Autodesk Fusion 360 part; units mm, degrees
(part 4 of 9)
  arc A178 (-216.55, 3.525) -> (-215.55, 2.525) centre (-215.55, 3.525) ccw
  line L174 (-216.55, 3.525) -> (-216.55, 15.525)
  arc A179 (-215.55, 16.525) -> (-216.55, 15.525) centre (-215.55, 15.525) ccw
  line L175 (-215.55, 16.525) -> (-203.55, 16.525)
  arc A180 (-202.55, 15.525) -> (-203.55, 16.525) centre (-203.55, 15.525) ccw
  line L176 (-243.0312, 53.625) -> (-243.0312, 41.625)
  arc A181 (-244.0312, 40.625) -> (-243.0313, 41.625) centre (-244.0313, 41.625) ccw
  line L177 (-244.0312, 40.625) -> (-256.0312, 40.625)
  arc A182 (-257.0312, 41.625) -> (-256.0312, 40.625) centre (-256.0312, 41.625) ccw
  line L178 (-257.0312, 41.625) -> (-257.0312, 53.625)
  arc A183 (-256.0312, 54.625) -> (-257.0312, 53.625) centre (-256.0312, 53.625) ccw
  line L179 (-256.0312, 54.625) -> (-244.0312, 54.625)
  arc A184 (-243.0313, 53.625) -> (-244.0312, 54.625) centre (-244.0312, 53.625) ccw
  arc A185 (-263.7, 57.15) -> (-266.7, 54.15) centre (-263.7, 54.15) ccw
  line L180 (-266.7, 54.15) -> (-266.7, 3)
  arc A186 (-266.7, 3) -> (-263.7, 0) centre (-263.7, 3) ccw
  line L181 (-263.7, 0) -> (-3, 0)
  arc A187 (-3, 0) -> (0, 3) centre (-3, 3) ccw
  line L182 (0, 3) -> (0, 54.15)
  arc A188 (0, 54.15) -> (-3, 57.15) centre (-3, 54.15) ccw
  line L183 (-3, 57.15) -> (-8.525, 57.15)
  arc A189 (-9.525, 58.15) -> (-8.525, 57.15) centre (-8.525, 58.15) ccw
  line L184 (-9.525, 58.15) -> (-9.525, 73.2)
  arc A190 (-9.525, 73.2) -> (-12.525, 76.2) centre (-12.525, 73.2) ccw
  line L185 (-12.525, 76.2) -> (-239.8875, 76.2)
  arc A191 (-239.8875, 76.2) -> (-242.8875, 73.2) centre (-239.8875, 73.2) ccw
  line L186 (-242.8875, 73.2) -> (-242.8875, 58.15)
  arc A192 (-243.8875, 57.15) -> (-242.8875, 58.15) centre (-243.8875, 58.15) ccw
  line L187 (-243.8875, 57.15) -> (-263.7, 57.15)
  line L188 (-47.625, 9.525) -> (-47.625, 6)
  line L189 (-47.625, 7.025) -> (-51.7449, 7.025)
  line L190 (-51.7449, 7.025) -> (-44, 7.025)
  line L191 (-44, 7.025) -> (-52, 7.025)
  line L192 (-52, 7.025) -> (-52, 12.025)
  line L193 (-52, 12.025) -> (-44, 12.025)
  line L194 (-44, 12.025) -> (-44, 7.025)
  dimension "d102" = 5
  constraint coincident A0.centre L188.start
  constraint vertical L188
  constraint coincident L188 L189.start
  constraint coincident A0 L189.start
  constraint tangent A0 L189
  constraint parallel L189 L190
  constraint horizontal L191
  constraint vertical L192
  constraint horizontal L193
  constraint vertical L194
  measures "d102" distance of L190.end L193.end
extrude "Extrude5" cut sketch "Sketch6" against normal blind 1.5 contours A0 L140 L189 L190 L191 L193 | A0 L47 L190 L191 L193
sketch "Sketch7" plane through (0, 0, 0) normal (0, -1, 0) x (1, 0, 0)
  circle A0 centre (47.625, 9.525) radius 1.25
  circle A1 centre (220.025, 66.675) radius 1.25
  circle A2 centre (245.269, 9.525) radius 1.25
  circle A3 centre (128.588, 37.025) radius 1.25
  circle A4 centre (32.525, 66.675) radius 1.25
  line L0 (162.7375, 59.675) -> (132.5375, 59.675)
  arc A5 (131.5375, 60.675) -> (132.5375, 59.675) centre (132.5375, 60.675) ccw
  line L1 (131.5375, 60.675) -> (131.5375, 72.675)
  arc A6 (132.5375, 73.675) -> (131.5375, 72.675) centre (132.5375, 72.675) ccw
  line L2 (132.5375, 73.675) -> (162.7375, 73.675)
  arc A7 (163.7375, 72.675) -> (162.7375, 73.675) centre (162.7375, 72.675) ccw
  line L3 (163.7375, 72.675) -> (163.7375, 60.675)
  arc A8 (162.7375, 59.675) -> (163.7375, 60.675) centre (162.7375, 60.675) ccw
  line L4 (36.5313, 40.625) -> (6.3312, 40.625)
  arc A9 (5.3312, 41.625) -> (6.3312, 40.625) centre (6.3312, 41.625) ccw
  line L5 (5.3312, 41.625) -> (5.3313, 53.625)
  arc A10 (6.3313, 54.625) -> (5.3312, 53.625) centre (6.3312, 53.625) ccw
  line L6 (6.3313, 54.625) -> (36.5312, 54.625)
  arc A11 (37.5313, 53.625) -> (36.5313, 54.625) centre (36.5313, 53.625) ccw
  line L7 (37.5312, 53.625) -> (37.5312, 41.625)
  arc A12 (36.5313, 40.625) -> (37.5313, 41.625) centre (36.5313, 41.625) ccw
  line L8 (92.0563, 73.675) -> (122.2563, 73.675)
  arc A13 (123.2563, 72.675) -> (122.2563, 73.675) centre (122.2563, 72.675) ccw
  line L9 (123.2563, 72.675) -> (123.2563, 60.675)
  arc A14 (122.2563, 59.675) -> (123.2563, 60.675) centre (122.2563, 60.675) ccw
  line L10 (122.2563, 59.675) -> (92.0563, 59.675)
  arc A15 (91.0563, 60.675) -> (92.0563, 59.675) centre (92.0563, 60.675) ccw
  line L11 (91.0563, 60.675) -> (91.0563, 72.675)
  arc A16 (92.0563, 73.675) -> (91.0563, 72.675) centre (92.0563, 72.675) ccw
  line L12 (230.1688, 35.575) -> (260.3688, 35.575)
  arc A17 (261.3688, 34.575) -> (260.3688, 35.575) centre (260.3687, 34.575) ccw
  line L13 (261.3688, 34.575) -> (261.3688, 22.575)
  arc A18 (260.3688, 21.575) -> (261.3688, 22.575) centre (260.3688, 22.575) ccw
  line L14 (260.3688, 21.575) -> (230.1688, 21.575)
  arc A19 (229.1688, 22.575) -> (230.1688, 21.575) centre (230.1688, 22.575) ccw
  line L15 (229.1688, 22.575) -> (229.1688, 34.575)
  arc A20 (230.1688, 35.575) -> (229.1688, 34.575) centre (230.1688, 34.575) ccw
  line L16 (250.175, 3.525) -> (250.175, 15.525)
  arc A21 (251.175, 16.525) -> (250.175, 15.525) centre (251.175, 15.525) ccw
  line L17 (251.175, 16.525) -> (263.175, 16.525)
  arc A22 (264.175, 15.525) -> (263.175, 16.525) centre (263.175, 15.525) ccw
  line L18 (264.175, 15.525) -> (264.175, 3.525)
  arc A23 (263.175, 2.525) -> (264.175, 3.525) centre (263.175, 3.525) ccw
  line L19 (263.175, 2.525) -> (251.175, 2.525)
  arc A24 (250.175, 3.525) -> (251.175, 2.525) centre (251.175, 3.525) ccw
  line L20 (216.8375, 41.625) -> (216.8375, 53.625)
  arc A25 (217.8375, 54.625) -> (216.8375, 53.625) centre (217.8375, 53.625) ccw
  line L21 (217.8375, 54.625) -> (229.8375, 54.625)
  arc A26 (230.8375, 53.625) -> (229.8375, 54.625) centre (229.8375, 53.625) ccw
  line L22 (230.8375, 53.625) -> (230.8375, 41.625)
  arc A27 (229.8375, 40.625) -> (230.8375, 41.625) centre (229.8375, 41.625) ccw
  line L23 (229.8375, 40.625) -> (217.8375, 40.625)
  arc A28 (216.8375, 41.625) -> (217.8375, 40.625) centre (217.8375, 41.625) ccw
  line L24 (188.2625, 22.575) -> (188.2625, 34.575)
  arc A29 (189.2625, 35.575) -> (188.2625, 34.575) centre (189.2625, 34.575) ccw
  line L25 (189.2625, 35.575) -> (201.2625, 35.575)
  arc A30 (202.2625, 34.575) -> (201.2625, 35.575) centre (201.2625, 34.575) ccw
  line L26 (202.2625, 34.575) -> (202.2625, 22.575)
  arc A31 (201.2625, 21.575) -> (202.2625, 22.575) centre (201.2625, 22.575) ccw
  line L27 (201.2625, 21.575) -> (189.2625, 21.575)
  arc A32 (188.2625, 22.575) -> (189.2625, 21.575) centre (189.2625, 22.575) ccw
  line L28 (178.7375, 41.625) -> (178.7375, 53.625)
  arc A33 (179.7375, 54.625) -> (178.7375, 53.625) centre (179.7375, 53.625) ccw
  line L29 (179.7375, 54.625) -> (191.7375, 54.625)
  arc A34 (192.7375, 53.625) -> (191.7375, 54.625) centre (191.7375, 53.625) ccw
  line L30 (192.7375, 53.625) -> (192.7375, 41.625)
  arc A35 (191.7375, 40.625) -> (192.7375, 41.625) centre (191.7375, 41.625) ccw
  line L31 (191.7375, 40.625) -> (179.7375, 40.625)
  arc A36 (178.7375, 41.625) -> (179.7375, 40.625) centre (179.7375, 41.625) ccw
  line L32 (140.6375, 41.625) -> (140.6375, 53.625)
  arc A37 (141.6375, 54.625) -> (140.6375, 53.625) centre (141.6375, 53.625) ccw
  line L33 (141.6375, 54.625) -> (153.6375, 54.625)
  arc A38 (154.6375, 53.625) -> (153.6375, 54.625) centre (153.6375, 53.625) ccw
  line L34 (154.6375, 53.625) -> (154.6375, 41.625)
  arc A39 (153.6375, 40.625) -> (154.6375, 41.625) centre (153.6375, 41.625) ccw
  line L35 (153.6375, 40.625) -> (141.6375, 40.625)
  arc A40 (140.6375, 41.625) -> (141.6375, 40.625) centre (141.6375, 41.625) ccw
  line L36 (131.1125, 22.575) -> (131.1125, 34.575)
  arc A41 (132.1125, 35.575) -> (131.1125, 34.575) centre (132.1125, 34.575) ccw
  line L37 (132.1125, 35.575) -> (144.1125, 35.575)
  arc A42 (145.1125, 34.575) -> (144.1125, 35.575) centre (144.1125, 34.575) ccw
  line L38 (145.1125, 34.575) -> (145.1125, 22.575)
  arc A43 (144.1125, 21.575) -> (145.1125, 22.575) centre (144.1125, 22.575) ccw
  line L39 (144.1125, 21.575) -> (132.1125, 21.575)
  arc A44 (131.1125, 22.575) -> (132.1125, 21.575) centre (132.1125, 22.575) ccw
  line L40 (107.3, 3.525) -> (107.3, 15.525)
  arc A45 (108.3, 16.525) -> (107.3, 15.525) centre (108.3, 15.525) ccw
  line L41 (108.3, 16.525) -> (120.3, 16.525)
  arc A46 (121.3, 15.525) -> (120.3, 16.525) centre (120.3, 15.525) ccw
  line L42 (121.3, 15.525) -> (121.3, 3.525)
  arc A47 (120.3, 2.525) -> (121.3, 3.525) centre (120.3, 3.525) ccw
  line L43 (120.3, 2.525) -> (108.3, 2.525)
  arc A48 (107.3, 3.525) -> (108.3, 2.525) centre (108.3, 3.525) ccw
  line L44 (69.2, 3.525) -> (69.2, 15.525)
  arc A49 (70.2, 16.525) -> (69.2, 15.525) centre (70.2, 15.525) ccw
  line L45 (70.2, 16.525) -> (82.2, 16.525)
  arc A50 (83.2, 15.525) -> (82.2, 16.525) centre (82.2, 15.525) ccw
  line L46 (83.2, 15.525) -> (83.2, 3.525)
  arc A51 (82.2, 2.525) -> (83.2, 3.525) centre (82.2, 3.525) ccw
  line L47 (82.2, 2.525) -> (70.2, 2.525)
  arc A52 (69.2, 3.525) -> (70.2, 2.525) centre (70.2, 3.525) ccw
  line L48 (45.3875, 41.625) -> (45.3875, 53.625)
  arc A53 (46.3875, 54.625) -> (45.3875, 53.625) centre (46.3875, 53.625) ccw
  line L49 (46.3875, 54.625) -> (58.3875, 54.625)
  arc A54 (59.3875, 53.625) -> (58.3875, 54.625) centre (58.3875, 53.625) ccw
  line L50 (59.3875, 53.625) -> (59.3875, 41.625)
  arc A55 (58.3875, 40.625) -> (59.3875, 41.625) centre (58.3875, 41.625) ccw
  line L51 (58.3875, 40.625) -> (46.3875, 40.625)
  arc A56 (45.3875, 41.625) -> (46.3875, 40.625) centre (46.3875, 41.625) ccw
  line L52 (9.6687, 22.575) -> (9.6688, 34.575)
  arc A57 (10.6687, 35.575) -> (9.6687, 34.575) centre (10.6688, 34.575) ccw
  line L53 (10.6687, 35.575) -> (22.6688, 35.575)
  arc A58 (23.6687, 34.575) -> (22.6687, 35.575) centre (22.6687, 34.575) ccw
  line L54 (23.6687, 34.575) -> (23.6688, 22.575)
  arc A59 (22.6687, 21.575) -> (23.6688, 22.575) centre (22.6687, 22.575) ccw
  line L55 (22.6688, 21.575) -> (10.6688, 21.575)
  arc A60 (9.6687, 22.575) -> (10.6687, 21.575) centre (10.6688, 22.575) ccw
  line L56 (32.1, 16.525) -> (44.1, 16.525)
  arc A61 (45.1, 15.525) -> (44.1, 16.525) centre (44.1, 15.525) ccw
  line L57 (45.1, 15.525) -> (45.1, 3.525)
  arc A62 (44.1, 2.525) -> (45.1, 3.525) centre (44.1, 3.525) ccw
  line L58 (44.1, 2.525) -> (32.1, 2.525)
  arc A63 (31.1, 3.525) -> (32.1, 2.525) centre (32.1, 3.525) ccw
  line L59 (31.1, 3.525) -> (31.1, 15.525)
  arc A64 (32.1, 16.525) -> (31.1, 15.525) centre (32.1, 15.525) ccw
  line L60 (40.625, 60.675) -> (40.625, 72.675)
  arc A65 (41.625, 73.675) -> (40.625, 72.675) centre (41.625, 72.675) ccw
  line L61 (41.625, 73.675) -> (53.625, 73.675)
  arc A66 (54.625, 72.675) -> (53.625, 73.675) centre (53.625, 72.675) ccw
  line L62 (54.625, 72.675) -> (54.625, 60.675)
  arc A67 (53.625, 59.675) -> (54.625, 60.675) centre (53.625, 60.675) ccw
  line L63 (53.625, 59.675) -> (41.625, 59.675)
  arc A68 (40.625, 60.675) -> (41.625, 59.675) centre (41.625, 60.675) ccw
  line L64 (54.9125, 22.575) -> (54.9125, 34.575)
  arc A69 (55.9125, 35.575) -> (54.9125, 34.575) centre (55.9125, 34.575) ccw
  line L65 (55.9125, 35.575) -> (67.9125, 35.575)
  arc A70 (68.9125, 34.575) -> (67.9125, 35.575) centre (67.9125, 34.575) ccw
  line L66 (68.9125, 34.575) -> (68.9125, 22.575)
  arc A71 (67.9125, 21.575) -> (68.9125, 22.575) centre (67.9125, 22.575) ccw
  line L67 (67.9125, 21.575) -> (55.9125, 21.575)
  arc A72 (54.9125, 22.575) -> (55.9125, 21.575) centre (55.9125, 22.575) ccw
  line L68 (66.8188, 60.675) -> (66.8188, 72.675)
  arc A73 (67.8188, 73.675) -> (66.8188, 72.675) centre (67.8188, 72.675) ccw
  line L69 (67.8188, 73.675) -> (79.8188, 73.675)
  arc A74 (80.8188, 72.675) -> (79.8188, 73.675) centre (79.8188, 72.675) ccw
  line L70 (80.8187, 72.675) -> (80.8187, 60.675)
  arc A75 (79.8188, 59.675) -> (80.8188, 60.675) centre (79.8188, 60.675) ccw
  line L71 (79.8188, 59.675) -> (67.8188, 59.675)
  arc A76 (66.8188, 60.675) -> (67.8188, 59.675) centre (67.8188, 60.675) ccw
  line L72 (88.25, 3.525) -> (88.25, 15.525)
  arc A77 (89.25, 16.525) -> (88.25, 15.525) centre (89.25, 15.525) ccw
  line L73 (89.25, 16.525) -> (101.25, 16.525)
  arc A78 (102.25, 15.525) -> (101.25, 16.525) centre (101.25, 15.525) ccw
  line L74 (102.25, 15.525) -> (102.25, 3.525)
  arc A79 (101.25, 2.525) -> (102.25, 3.525) centre (101.25, 3.525) ccw
  line L75 (101.25, 2.525) -> (89.25, 2.525)
  arc A80 (88.25, 3.525) -> (89.25, 2.525) centre (89.25, 3.525) ccw
  line L76 (121.5875, 41.625) -> (121.5875, 53.625)
  arc A81 (122.5875, 54.625) -> (121.5875, 53.625) centre (122.5875, 53.625) ccw
  line L77 (122.5875, 54.625) -> (134.5875, 54.625)
  arc A82 (135.5875, 53.625) -> (134.5875, 54.625) centre (134.5875, 53.625) ccw
  line L78 (135.5875, 53.625) -> (135.5875, 41.625)
  arc A83 (134.5875, 40.625) -> (135.5875, 41.625) centre (134.5875, 41.625) ccw
  line L79 (134.5875, 40.625) -> (122.5875, 40.625)
  arc A84 (121.5875, 41.625) -> (122.5875, 40.625) centre (122.5875, 41.625) ccw
  line L80 (150.1625, 22.575) -> (150.1625, 34.575)
  arc A85 (151.1625, 35.575) -> (150.1625, 34.575) centre (151.1625, 34.575) ccw
  line L81 (151.1625, 35.575) -> (163.1625, 35.575)
  arc A86 (164.1625, 34.575) -> (163.1625, 35.575) centre (163.1625, 34.575) ccw
  line L82 (164.1625, 34.575) -> (164.1625, 22.575)
  arc A87 (163.1625, 21.575) -> (164.1625, 22.575) centre (163.1625, 22.575) ccw
  line L83 (163.1625, 21.575) -> (151.1625, 21.575)
  arc A88 (150.1625, 22.575) -> (151.1625, 21.575) centre (151.1625, 22.575) ccw
  line L84 (171.5937, 60.675) -> (171.5938, 72.675)
  arc A89 (172.5937, 73.675) -> (171.5938, 72.675) centre (172.5937, 72.675) ccw
  line L85 (172.5938, 73.675) -> (184.5938, 73.675)
  arc A90 (185.5937, 72.675) -> (184.5938, 73.675) centre (184.5937, 72.675) ccw
  line L86 (185.5937, 72.675) -> (185.5937, 60.675)
  arc A91 (184.5938, 59.675) -> (185.5938, 60.675) centre (184.5938, 60.675) ccw
  line L87 (184.5938, 59.675) -> (172.5937, 59.675)
  arc A92 (171.5937, 60.675) -> (172.5938, 59.675) centre (172.5937, 60.675) ccw
  line L88 (183.5, 3.525) -> (183.5, 15.525)
  arc A93 (184.5, 16.525) -> (183.5, 15.525) centre (184.5, 15.525) ccw
  line L89 (184.5, 16.525) -> (196.5, 16.525)
  arc A94 (197.5, 15.525) -> (196.5, 16.525) centre (196.5, 15.525) ccw
  line L90 (197.5, 15.525) -> (197.5, 3.525)
  arc A95 (196.5, 2.525) -> (197.5, 3.525) centre (196.5, 3.525) ccw
  line L91 (196.5, 2.525) -> (184.5, 2.525)
  arc A96 (183.5, 3.525) -> (184.5, 2.525) centre (184.5, 3.525) ccw
  line L92 (223.9812, 60.675) -> (223.9813, 72.675)
  arc A97 (224.9813, 73.675) -> (223.9813, 72.675) centre (224.9812, 72.675) ccw
  line L93 (224.9813, 73.675) -> (236.9813, 73.675)
  arc A98 (237.9812, 72.675) -> (236.9813, 73.675) centre (236.9813, 72.675) ccw
  line L94 (237.9812, 72.675) -> (237.9813, 60.675)
  arc A99 (236.9813, 59.675) -> (237.9813, 60.675) centre (236.9813, 60.675) ccw
  line L95 (236.9813, 59.675) -> (224.9813, 59.675)
  arc A100 (223.9813, 60.675) -> (224.9813, 59.675) centre (224.9812, 60.675) ccw
  line L96 (226.3625, 3.525) -> (226.3625, 15.525)
  arc A101 (227.3625, 16.525) -> (226.3625, 15.525) centre (227.3625, 15.525) ccw
  line L97 (227.3625, 16.525) -> (239.3625, 16.525)
  arc A102 (240.3625, 15.525) -> (239.3625, 16.525) centre (239.3625, 15.525) ccw
  line L98 (240.3625, 15.525) -> (240.3625, 3.525)
  arc A103 (239.3625, 2.525) -> (240.3625, 3.525) centre (239.3625, 3.525) ccw
  line L99 (239.3625, 2.525) -> (227.3625, 2.525)
  arc A104 (226.3625, 3.525) -> (227.3625, 2.525) centre (227.3625, 3.525) ccw
  line L100 (207.3125, 22.575) -> (207.3125, 34.575)
  arc A105 (208.3125, 35.575) -> (207.3125, 34.575) centre (208.3125, 34.575) ccw
  line L101 (208.3125, 35.575) -> (220.3125, 35.575)
  arc A106 (221.3125, 34.575) -> (220.3125, 35.575) centre (220.3125, 34.575) ccw
  line L102 (221.3125, 34.575) -> (221.3125, 22.575)
  arc A107 (220.3125, 21.575) -> (221.3125, 22.575) centre (220.3125, 22.575) ccw
  line L103 (220.3125, 21.575) -> (208.3125, 21.575)
  arc A108 (207.3125, 22.575) -> (208.3125, 21.575) centre (208.3125, 22.575) ccw
  line L104 (197.7875, 41.625) -> (197.7875, 53.625)
  arc A109 (198.7875, 54.625) -> (197.7875, 53.625) centre (198.7875, 53.625) ccw
  line L105 (198.7875, 54.625) -> (210.7875, 54.625)
  arc A110 (211.7875, 53.625) -> (210.7875, 54.625) centre (210.7875, 53.625) ccw
  line L106 (211.7875, 53.625) -> (211.7875, 41.625)
  arc A111 (210.7875, 40.625) -> (211.7875, 41.625) centre (210.7875, 41.625) ccw
  line L107 (210.7875, 40.625) -> (198.7875, 40.625)
  arc A112 (197.7875, 41.625) -> (198.7875, 40.625) centre (198.7875, 41.625) ccw
  line L108 (169.2125, 22.575) -> (169.2125, 34.575)
  arc A113 (170.2125, 35.575) -> (169.2125, 34.575) centre (170.2125, 34.575) ccw
  line L109 (170.2125, 35.575) -> (182.2125, 35.575)
  arc A114 (183.2125, 34.575) -> (182.2125, 35.575) centre (182.2125, 34.575) ccw
  line L110 (183.2125, 34.575) -> (183.2125, 22.575)
  arc A115 (182.2125, 21.575) -> (183.2125, 22.575) centre (182.2125, 22.575) ccw
  line L111 (182.2125, 21.575) -> (170.2125, 21.575)
  arc A116 (169.2125, 22.575) -> (170.2125, 21.575) centre (170.2125, 22.575) ccw
  line L112 (126.35, 3.525) -> (126.35, 15.525)
  arc A117 (127.35, 16.525) -> (126.35, 15.525) centre (127.35, 15.525) ccw
  line L113 (127.35, 16.525) -> (139.35, 16.525)
  arc A118 (140.35, 15.525) -> (139.35, 16.525) centre (139.35, 15.525) ccw
  line L114 (140.35, 15.525) -> (140.35, 3.525)
  arc A119 (139.35, 2.525) -> (140.35, 3.525) centre (139.35, 3.525) ccw
  line L115 (139.35, 2.525) -> (127.35, 2.525)
  arc A120 (126.35, 3.525) -> (127.35, 2.525) centre (127.35, 3.525) ccw
  line L116 (112.0625, 22.575) -> (112.0625, 34.575)
  arc A121 (113.0625, 35.575) -> (112.0625, 34.575) centre (113.0625, 34.575) ccw
  line L117 (113.0625, 35.575) -> (125.0625, 35.575)
  arc A122 (126.0625, 34.575) -> (125.0625, 35.575) centre (125.0625, 34.575) ccw
  line L118 (126.0625, 34.575) -> (126.0625, 22.575)
  arc A123 (125.0625, 21.575) -> (126.0625, 22.575) centre (125.0625, 22.575) ccw
  line L119 (125.0625, 21.575) -> (113.0625, 21.575)
  arc A124 (112.0625, 22.575) -> (113.0625, 21.575) centre (113.0625, 22.575) ccw
  line L120 (83.4875, 41.625) -> (83.4875, 53.625)
  arc A125 (84.4875, 54.625) -> (83.4875, 53.625) centre (84.4875, 53.625) ccw
  line L121 (84.4875, 54.625) -> (96.4875, 54.625)
  arc A126 (97.4875, 53.625) -> (96.4875, 54.625) centre (96.4875, 53.625) ccw
  line L122 (97.4875, 53.625) -> (97.4875, 41.625)
  arc A127 (96.4875, 40.625) -> (97.4875, 41.625) centre (96.4875, 41.625) ccw
  line L123 (96.4875, 40.625) -> (84.4875, 40.625)
  arc A128 (83.4875, 41.625) -> (84.4875, 40.625) centre (84.4875, 41.625) ccw
  line L124 (73.9625, 22.575) -> (73.9625, 34.575)
  arc A129 (74.9625, 35.575) -> (73.9625, 34.575) centre (74.9625, 34.575) ccw
  line L125 (74.9625, 35.575) -> (86.9625, 35.575)
  arc A130 (87.9625, 34.575) -> (86.9625, 35.575) centre (86.9625, 34.575) ccw
  line L126 (87.9625, 34.575) -> (87.9625, 22.575)
  arc A131 (86.9625, 21.575) -> (87.9625, 22.575) centre (86.9625, 22.575) ccw
  line L127 (86.9625, 21.575) -> (74.9625, 21.575)
  arc A132 (73.9625, 22.575) -> (74.9625, 21.575) centre (74.9625, 22.575) ccw
  line L128 (35.8625, 22.575) -> (35.8625, 34.575)
  arc A133 (36.8625, 35.575) -> (35.8625, 34.575) centre (36.8625, 34.575) ccw
  line L129 (36.8625, 35.575) -> (48.8625, 35.575)
  arc A134 (49.8625, 34.575) -> (48.8625, 35.575) centre (48.8625, 34.575) ccw
  line L130 (49.8625, 34.575) -> (49.8625, 22.575)
  arc A135 (48.8625, 21.575) -> (49.8625, 22.575) centre (48.8625, 22.575) ccw
  line L131 (48.8625, 21.575) -> (36.8625, 21.575)
  arc A136 (35.8625, 22.575) -> (36.8625, 21.575) centre (36.8625, 22.575) ccw
  line L132 (7.2875, 3.525) -> (7.2875, 15.525)
  arc A137 (8.2875, 16.525) -> (7.2875, 15.525) centre (8.2875, 15.525) ccw
  line L133 (8.2875, 16.525) -> (20.2875, 16.525)
  arc A138 (21.2875, 15.525) -> (20.2875, 16.525) centre (20.2875, 15.525) ccw
  line L134 (21.2875, 15.525) -> (21.2875, 3.525)
  arc A139 (20.2875, 2.525) -> (21.2875, 3.525) centre (20.2875, 3.525) ccw
  line L135 (20.2875, 2.525) -> (8.2875, 2.525)
  arc A140 (7.2875, 3.525) -> (8.2875, 2.525) centre (8.2875, 3.525) ccw
  line L136 (14.4313, 60.675) -> (14.4313, 72.675)
  arc A141 (15.4313, 73.675) -> (14.4313, 72.675) centre (15.4313, 72.675) ccw
  line L137 (15.4313, 73.675) -> (27.4313, 73.675)
  arc A142 (28.4312, 72.675) -> (27.4313, 73.675) centre (27.4312, 72.675) ccw
  line L138 (28.4312, 72.675) -> (28.4313, 60.675)
  arc A143 (27.4313, 59.675) -> (28.4313, 60.675) centre (27.4313, 60.675) ccw
  line L139 (27.4313, 59.675) -> (15.4313, 59.675)
  arc A144 (14.4313, 60.675) -> (15.4313, 59.675) centre (15.4312, 60.675) ccw
  line L140 (50.15, 3.525) -> (50.15, 15.525)
  arc A145 (51.15, 16.525) -> (50.15, 15.525) centre (51.15, 15.525) ccw
  line L141 (51.15, 16.525) -> (63.15, 16.525)
  arc A146 (64.15, 15.525) -> (63.15, 16.525) centre (63.15, 15.525) ccw
  line L142 (64.15, 15.525) -> (64.15, 3.525)
  arc A147 (63.15, 2.525) -> (64.15, 3.525) centre (63.15, 3.525) ccw
  line L143 (63.15, 2.525) -> (51.15, 2.525)
  arc A148 (50.15, 3.525) -> (51.15, 2.525) centre (51.15, 3.525) ccw
  line L144 (64.4375, 41.625) -> (64.4375, 53.625)
  arc A149 (65.4375, 54.625) -> (64.4375, 53.625) centre (65.4375, 53.625) ccw
  line L145 (65.4375, 54.625) -> (77.4375, 54.625)
  arc A150 (78.4375, 53.625) -> (77.4375, 54.625) centre (77.4375, 53.625) ccw
  line L146 (78.4375, 53.625) -> (78.4375, 41.625)
  arc A151 (77.4375, 40.625) -> (78.4375, 41.625) centre (77.4375, 41.625) ccw
  line L147 (77.4375, 40.625) -> (65.4375, 40.625)
  arc A152 (64.4375, 41.625) -> (65.4375, 40.625) centre (65.4375, 41.625) ccw
  line L148 (93.0125, 22.575) -> (93.0125, 34.575)
  arc A153 (94.0125, 35.575) -> (93.0125, 34.575) centre (94.0125, 34.575) ccw
  line L149 (94.0125, 35.575) -> (106.0125, 35.575)
  arc A154 (107.0125, 34.575) -> (106.0125, 35.575) centre (106.0125, 34.575) ccw
  line L150 (107.0125, 34.575) -> (107.0125, 22.575)
  arc A155 (106.0125, 21.575) -> (107.0125, 22.575) centre (106.0125, 22.575) ccw
  line L151 (106.0125, 21.575) -> (94.0125, 21.575)
  arc A156 (93.0125, 22.575) -> (94.0125, 21.575) centre (94.0125, 22.575) ccw
  line L152 (102.5375, 41.625) -> (102.5375, 53.625)
  arc A157 (103.5375, 54.625) -> (102.5375, 53.625) centre (103.5375, 53.625) ccw
  line L153 (103.5375, 54.625) -> (115.5375, 54.625)
  arc A158 (116.5375, 53.625) -> (115.5375, 54.625) centre (115.5375, 53.625) ccw
  line L154 (116.5375, 53.625) -> (116.5375, 41.625)
  arc A159 (115.5375, 40.625) -> (116.5375, 41.625) centre (115.5375, 41.625) ccw
  line L155 (115.5375, 40.625) -> (103.5375, 40.625)
  arc A160 (102.5375, 41.625) -> (103.5375, 40.625) centre (103.5375, 41.625) ccw
  line L156 (145.4, 3.525) -> (145.4, 15.525)
  arc A161 (146.4, 16.525) -> (145.4, 15.525) centre (146.4, 15.525) ccw
  line L157 (146.4, 16.525) -> (158.4, 16.525)
  arc A162 (159.4, 15.525) -> (158.4, 16.525) centre (158.4, 15.525) ccw
  line L158 (159.4, 15.525) -> (159.4, 3.525)
  arc A163 (158.4, 2.525) -> (159.4, 3.525) centre (158.4, 3.525) ccw
  line L159 (158.4, 2.525) -> (146.4, 2.525)
  arc A164 (145.4, 3.525) -> (146.4, 2.525) centre (146.4, 3.525) ccw
  line L160 (159.6875, 41.625) -> (159.6875, 53.625)
  arc A165 (160.6875, 54.625) -> (159.6875, 53.625) centre (160.6875, 53.625) ccw
  line L161 (160.6875, 54.625) -> (172.6875, 54.625)
  arc A166 (173.6875, 53.625) -> (172.6875, 54.625) centre (172.6875, 53.625) ccw
  line L162 (173.6875, 53.625) -> (173.6875, 41.625)
  arc A167 (172.6875, 40.625) -> (173.6875, 41.625) centre (172.6875, 41.625) ccw
  line L163 (172.6875, 40.625) -> (160.6875, 40.625)
  arc A168 (159.6875, 41.625) -> (160.6875, 40.625) centre (160.6875, 41.625) ccw
  line L164 (164.45, 3.525) -> (164.45, 15.525)
  arc A169 (165.45, 16.525) -> (164.45, 15.525) centre (165.45, 15.525) ccw
  line L165 (165.45, 16.525) -> (177.45, 16.525)
  arc A170 (178.45, 15.525) -> (177.45, 16.525) centre (177.45, 15.525) ccw
  line L166 (178.45, 15.525) -> (178.45, 3.525)
  arc A171 (177.45, 2.525) -> (178.45, 3.525) centre (177.45, 3.525) ccw
  line L167 (177.45, 2.525) -> (165.45, 2.525)
  arc A172 (164.45, 3.525) -> (165.45, 2.525) centre (165.45, 3.525) ccw
  line L168 (197.7875, 60.675) -> (197.7875, 72.675)
  arc A173 (198.7875, 73.675) -> (197.7875, 72.675) centre (198.7875, 72.675) ccw
  line L169 (198.7875, 73.675) -> (210.7875, 73.675)
  arc A174 (211.7875, 72.675) -> (210.7875, 73.675) centre (210.7875, 72.675) ccw
  line L170 (211.7875, 72.675) -> (211.7875, 60.675)
  arc A175 (210.7875, 59.675) -> (211.7875, 60.675) centre (210.7875, 60.675) ccw
  line L171 (210.7875, 59.675) -> (198.7875, 59.675)
  arc A176 (197.7875, 60.675) -> (198.7875, 59.675) centre (198.7875, 60.675) ccw
  line L172 (202.55, 3.525) -> (202.55, 15.525)
  arc A177 (203.55, 16.525) -> (202.55, 15.525) centre (203.55, 15.525) ccw
  line L173 (203.55, 16.525) -> (215.55, 16.525)
  arc A178 (216.55, 15.525) -> (215.55, 16.525) centre (215.55, 15.525) ccw
  line L174 (216.55, 15.525) -> (216.55, 3.525)
  arc A179 (215.55, 2.525) -> (216.55, 3.525) centre (215.55, 3.525) ccw
  line L175 (215.55, 2.525) -> (203.55, 2.525)
  arc A180 (202.55, 3.525) -> (203.55, 2.525) centre (203.55, 3.525) ccw
  line L176 (243.0312, 41.625) -> (243.0312, 53.625)
  arc A181 (244.0312, 54.625) -> (243.0313, 53.625) centre (244.0312, 53.625) ccw
  line L177 (244.0312, 54.625) -> (256.0312, 54.625)
  arc A182 (257.0312, 53.625) -> (256.0312, 54.625) centre (256.0312, 53.625) ccw
  line L178 (257.0312, 53.625) -> (257.0312, 41.625)
  arc A183 (256.0312, 40.625) -> (257.0312, 41.625) centre (256.0312, 41.625) ccw
  line L179 (256.0312, 40.625) -> (244.0312, 40.625)
  arc A184 (243.0312, 41.625) -> (244.0312, 40.625) centre (244.0313, 41.625) ccw
  arc A185 (266.7, 54.15) -> (263.7, 57.15) centre (263.7, 54.15) ccw
  line L180 (263.7, 57.15) -> (243.8875, 57.15)
  arc A186 (242.8875, 58.15) -> (243.8875, 57.15) centre (243.8875, 58.15) ccw
  line L181 (242.8875, 58.15) -> (242.8875, 73.2)
  arc A187 (242.8875, 73.2) -> (239.8875, 76.2) centre (239.8875, 73.2) ccw
  line L182 (239.8875, 76.2) -> (12.525, 76.2)
  arc A188 (12.525, 76.2) -> (9.525, 73.2) centre (12.525, 73.2) ccw
  line L183 (9.525, 73.2) -> (9.525, 58.15)
  arc A189 (8.525, 57.15) -> (9.525, 58.15) centre (8.525, 58.15) ccw
  line L184 (8.525, 57.15) -> (3, 57.15)
  arc A190 (3, 57.15) -> (0, 54.15) centre (3, 54.15) ccw
  line L185 (0, 54.15) -> (0, 3)
  arc A191 (0, 3) -> (3, 0) centre (3, 3) ccw
  line L186 (3, 0) -> (263.7, 0)
  arc A192 (263.7, 0) -> (266.7, 3) centre (263.7, 3) ccw
  line L187 (266.7, 3) -> (266.7, 54.15)
  line L188 (18.9312, 73.675) -> (23.9312, 73.675)
  line L189 (23.9312, 73.675) -> (23.9312, 74.675)
  line L190 (23.9312, 74.675) -> (18.9312, 74.675)
  line L191 (18.9312, 74.675) -> (18.9312, 73.675)
  line L192 (18.9313, 59.675) -> (23.9313, 59.675)
  line L193 (23.9313, 59.675) -> (23.9313, 58.675)
  line L194 (23.9313, 58.675) -> (18.9313, 58.675)
  line L195 (18.9313, 58.675) -> (18.9313, 59.675)
  line L196 (11.05, 73.2) -> (11.05, 58.15)
  arc A193 (8.525, 55.625) -> (11.05, 58.15) centre (8.525, 58.15) ccw
  line L197 (8.525, 55.625) -> (3, 55.625)
  arc A194 (3, 55.625) -> (1.525, 54.15) centre (3, 54.15) ccw
  line L198 (1.525, 54.15) -> (1.525, 3)
  arc A195 (1.525, 3) -> (3, 1.525) centre (3, 3) ccw
  line L199 (3, 1.525) -> (263.7, 1.525)
  arc A196 (263.7, 1.525) -> (265.175, 3) centre (263.7, 3) ccw
  line L200 (265.175, 3) -> (265.175, 54.15)
  arc A197 (265.175, 54.15) -> (263.7, 55.625) centre (263.7, 54.15) ccw
  line L201 (263.7, 55.625) -> (243.8875, 55.625)
  arc A198 (241.3625, 58.15) -> (243.8875, 55.625) centre (243.8875, 58.15) ccw
  line L202 (241.3625, 58.15) -> (241.3625, 73.2)
  arc A199 (241.3625, 73.2) -> (239.8875, 74.675) centre (239.8875, 73.2) ccw
  line L203 (239.8875, 74.675) -> (12.525, 74.675)
  arc A200 (12.525, 74.675) -> (11.05, 73.2) centre (12.525, 73.2) ccw
  dimension "d105" = 5
  dimension "d106" = 1
  dimension "d107" = 4.5
  dimension "d108" = 5
  dimension "d109" = 1
  dimension "d110" = 4.5
  dimension "d111" = 1.525
  constraint horizontal L188
  constraint vertical L189
  constraint horizontal L190
  constraint vertical L191
  constraint coincident L137 L188.start
  constraint horizontal L192
  constraint vertical L193
  constraint horizontal L194
  constraint vertical L195
  constraint coincident L139 L192.start
  measures "d105" distance of L188.start L188.end
  measures "d106" distance of L188.start L190.end
  measures "d107" distance of L138 L189
  measures "d108" distance of L192.start L192.end
  measures "d109" distance of L192.start L194.end
  measures "d110" distance of L138 L193
extrude "Extrude6" cut sketch "Sketch7" against normal blind 0.6 contours L136 A141 L137 A142 L138 A143 L139 A144 L189 L191 L193 L194 L195 L196 A193 L197 A194 L198 A195 L199 A196 L200 A197 L201 A198 L202 A199 L203 A200 | L139 L192 L193 L194 L195 | L137 L188 L189 L190 L191 L203
sketch "Sketch8" plane through (0, 0.6, 0) normal (0, -1, 0) x (1, 0, 0)
  arc A0 (65.4375, 54.625) -> (64.4375, 53.625) centre (65.4375, 53.625) ccw
  line L0 (65.4375, 54.625) -> (77.4375, 54.625)
  arc A1 (78.4375, 53.625) -> (77.4375, 54.625) centre (77.4375, 53.625) ccw
  line L1 (78.4375, 53.625) -> (78.4375, 41.625)
  arc A2 (77.4375, 40.625) -> (78.4375, 41.625) centre (77.4375, 41.625) ccw
  line L2 (77.4375, 40.625) -> (65.4375, 40.625)
  arc A3 (64.4375, 41.625) -> (65.4375, 40.625) centre (65.4375, 41.625) ccw
  line L3 (64.4375, 41.625) -> (64.4375, 53.625)
  arc A4 (198.7875, 73.675) -> (197.7875, 72.675) centre (198.7875, 72.675) ccw
  line L4 (198.7875, 73.675) -> (210.7875, 73.675)
  arc A5 (211.7875, 72.675) -> (210.7875, 73.675) centre (210.7875, 72.675) ccw
  line L5 (211.7875, 72.675) -> (211.7875, 60.675)
  arc A6 (210.7875, 59.675) -> (211.7875, 60.675) centre (210.7875, 60.675) ccw
  line L6 (210.7875, 59.675) -> (198.7875, 59.675)
  arc A7 (197.7875, 60.675) -> (198.7875, 59.675) centre (198.7875, 60.675) ccw
  line L7 (197.7875, 60.675) -> (197.7875, 72.675)
  arc A8 (244.0312, 54.625) -> (243.0313, 53.625) centre (244.0312, 53.625) ccw
  line L8 (244.0312, 54.625) -> (256.0312, 54.625)
  arc A9 (257.0312, 53.625) -> (256.0312, 54.625) centre (256.0312, 53.625) ccw
  line L9 (257.0312, 53.625) -> (257.0312, 41.625)
  arc A10 (256.0312, 40.625) -> (257.0312, 41.625) centre (256.0312, 41.625) ccw
  line L10 (256.0312, 40.625) -> (244.0312, 40.625)
  arc A11 (243.0313, 41.625) -> (244.0312, 40.625) centre (244.0312, 41.625) ccw
  line L11 (243.0312, 41.625) -> (243.0312, 53.625)
  arc A12 (14.4313, 60.675) -> (15.4313, 59.675) centre (15.4313, 60.675) ccw
  line L12 (14.4313, 60.675) -> (14.4313, 72.675)
  arc A13 (15.4313, 73.675) -> (14.4313, 72.675) centre (15.4313, 72.675) ccw
  line L13 (15.4313, 73.675) -> (27.4313, 73.675)
  arc A14 (28.4312, 72.675) -> (27.4313, 73.675) centre (27.4312, 72.675) ccw
  line L14 (28.4312, 72.675) -> (28.4313, 60.675)
  arc A15 (27.4313, 59.675) -> (28.4313, 60.675) centre (27.4313, 60.675) ccw
  line L15 (27.4313, 59.675) -> (15.4313, 59.675)
  arc A16 (165.45, 16.525) -> (164.45, 15.525) centre (165.45, 15.525) ccw
  line L16 (165.45, 16.525) -> (177.45, 16.525)
  arc A17 (178.45, 15.525) -> (177.45, 16.525) centre (177.45, 15.525) ccw
  line L17 (178.45, 15.525) -> (178.45, 3.525)
  arc A18 (177.45, 2.525) -> (178.45, 3.525) centre (177.45, 3.525) ccw
  line L18 (177.45, 2.525) -> (165.45, 2.525)
  arc A19 (164.45, 3.525) -> (165.45, 2.525) centre (165.45, 3.525) ccw
  line L19 (164.45, 3.525) -> (164.45, 15.525)
  arc A20 (67.8188, 73.675) -> (66.8188, 72.675) centre (67.8188, 72.675) ccw
  line L20 (67.8188, 73.675) -> (79.8188, 73.675)
  arc A21 (80.8188, 72.675) -> (79.8188, 73.675) centre (79.8188, 72.675) ccw
  line L21 (80.8187, 72.675) -> (80.8187, 60.675)
  arc A22 (79.8188, 59.675) -> (80.8188, 60.675) centre (79.8188, 60.675) ccw
  line L22 (79.8188, 59.675) -> (67.8188, 59.675)
  arc A23 (66.8188, 60.675) -> (67.8188, 59.675) centre (67.8188, 60.675) ccw
  line L23 (66.8188, 60.675) -> (66.8188, 72.675)
  arc A24 (261.3688, 34.575) -> (260.3688, 35.575) centre (260.3688, 34.575) ccw
  line L24 (261.3688, 34.575) -> (261.3688, 22.575)
  arc A25 (260.3688, 21.575) -> (261.3688, 22.575) centre (260.3688, 22.575) ccw
  line L25 (260.3688, 21.575) -> (230.1688, 21.575)
  arc A26 (229.1688, 22.575) -> (230.1688, 21.575) centre (230.1688, 22.575) ccw
  line L26 (229.1688, 22.575) -> (229.1688, 34.575)
  arc A27 (230.1688, 35.575) -> (229.1688, 34.575) centre (230.1688, 34.575) ccw
  line L27 (230.1688, 35.575) -> (260.3688, 35.575)
  arc A28 (184.5, 16.525) -> (183.5, 15.525) centre (184.5, 15.525) ccw
  line L28 (184.5, 16.525) -> (196.5, 16.525)
  arc A29 (197.5, 15.525) -> (196.5, 16.525) centre (196.5, 15.525) ccw
  line L29 (197.5, 15.525) -> (197.5, 3.525)
  arc A30 (196.5, 2.525) -> (197.5, 3.525) centre (196.5, 3.525) ccw
  line L30 (196.5, 2.525) -> (184.5, 2.525)
  arc A31 (183.5, 3.525) -> (184.5, 2.525) centre (184.5, 3.525) ccw
  line L31 (183.5, 3.525) -> (183.5, 15.525)
  arc A32 (45.1, 15.525) -> (44.1, 16.525) centre (44.1, 15.525) ccw
  line L32 (45.1, 15.525) -> (45.1, 3.525)
  arc A33 (44.1, 2.525) -> (45.1, 3.525) centre (44.1, 3.525) ccw
  line L33 (44.1, 2.525) -> (32.1, 2.525)
  arc A34 (31.1, 3.525) -> (32.1, 2.525) centre (32.1, 3.525) ccw
  line L34 (31.1, 3.525) -> (31.1, 15.525)
  arc A35 (32.1, 16.525) -> (31.1, 15.525) centre (32.1, 15.525) ccw
  line L35 (32.1, 16.525) -> (44.1, 16.525)
  arc A36 (55.9125, 35.575) -> (54.9125, 34.575) centre (55.9125, 34.575) ccw
  line L36 (55.9125, 35.575) -> (67.9125, 35.575)
  arc A37 (68.9125, 34.575) -> (67.9125, 35.575) centre (67.9125, 34.575) ccw
  line L37 (68.9125, 34.575) -> (68.9125, 22.575)
  arc A38 (67.9125, 21.575) -> (68.9125, 22.575) centre (67.9125, 22.575) ccw
  line L38 (67.9125, 21.575) -> (55.9125, 21.575)
  arc A39 (54.9125, 22.575) -> (55.9125, 21.575) centre (55.9125, 22.575) ccw
  line L39 (54.9125, 22.575) -> (54.9125, 34.575)
  arc A40 (46.3875, 54.625) -> (45.3875, 53.625) centre (46.3875, 53.625) ccw
  line L40 (46.3875, 54.625) -> (58.3875, 54.625)
  arc A41 (59.3875, 53.625) -> (58.3875, 54.625) centre (58.3875, 53.625) ccw
  line L41 (59.3875, 53.625) -> (59.3875, 41.625)
  arc A42 (58.3875, 40.625) -> (59.3875, 41.625) centre (58.3875, 41.625) ccw
  line L42 (58.3875, 40.625) -> (46.3875, 40.625)
  arc A43 (45.3875, 41.625) -> (46.3875, 40.625) centre (46.3875, 41.625) ccw
  line L43 (45.3875, 41.625) -> (45.3875, 53.625)
  arc A44 (70.2, 16.525) -> (69.2, 15.525) centre (70.2, 15.525) ccw
  line L44 (70.2, 16.525) -> (82.2, 16.525)
  arc A45 (83.2, 15.525) -> (82.2, 16.525) centre (82.2, 15.525) ccw
  line L45 (83.2, 15.525) -> (83.2, 3.525)
  arc A46 (82.2, 2.525) -> (83.2, 3.525) centre (82.2, 3.525) ccw
  line L46 (82.2, 2.525) -> (70.2, 2.525)
  arc A47 (69.2, 3.525) -> (70.2, 2.525) centre (70.2, 3.525) ccw
  line L47 (69.2, 3.525) -> (69.2, 15.525)
  arc A48 (10.6688, 35.575) -> (9.6688, 34.575) centre (10.6688, 34.575) ccw
  line L48 (10.6688, 35.575) -> (22.6687, 35.575)
  arc A49 (23.6687, 34.575) -> (22.6687, 35.575) centre (22.6687, 34.575) ccw
  line L49 (23.6687, 34.575) -> (23.6688, 22.575)
  arc A50 (22.6687, 21.575) -> (23.6688, 22.575) centre (22.6688, 22.575) ccw
  line L50 (22.6687, 21.575) -> (10.6688, 21.575)
  arc A51 (9.6687, 22.575) -> (10.6688, 21.575) centre (10.6687, 22.575) ccw
  line L51 (9.6687, 22.575) -> (9.6688, 34.575)
  arc A52 (172.5938, 73.675) -> (171.5938, 72.675) centre (172.5938, 72.675) ccw
  line L52 (172.5938, 73.675) -> (184.5938, 73.675)
  arc A53 (185.5937, 72.675) -> (184.5938, 73.675) centre (184.5937, 72.675) ccw
  line L53 (185.5937, 72.675) -> (185.5937, 60.675)
  arc A54 (184.5938, 59.675) -> (185.5937, 60.675) centre (184.5938, 60.675) ccw
  line L54 (184.5938, 59.675) -> (172.5937, 59.675)
  arc A55 (171.5938, 60.675) -> (172.5938, 59.675) centre (172.5938, 60.675) ccw
  line L55 (171.5937, 60.675) -> (171.5938, 72.675)
  arc A56 (151.1625, 35.575) -> (150.1625, 34.575) centre (151.1625, 34.575) ccw
  line L56 (151.1625, 35.575) -> (163.1625, 35.575)
  arc A57 (164.1625, 34.575) -> (163.1625, 35.575) centre (163.1625, 34.575) ccw
  line L57 (164.1625, 34.575) -> (164.1625, 22.575)
  arc A58 (163.1625, 21.575) -> (164.1625, 22.575) centre (163.1625, 22.575) ccw
  line L58 (163.1625, 21.575) -> (151.1625, 21.575)
  arc A59 (150.1625, 22.575) -> (151.1625, 21.575) centre (151.1625, 22.575) ccw
  line L59 (150.1625, 22.575) -> (150.1625, 34.575)
  arc A60 (89.25, 16.525) -> (88.25, 15.525) centre (89.25, 15.525) ccw
  line L60 (89.25, 16.525) -> (101.25, 16.525)
  arc A61 (102.25, 15.525) -> (101.25, 16.525) centre (101.25, 15.525) ccw
  line L61 (102.25, 15.525) -> (102.25, 3.525)
  arc A62 (101.25, 2.525) -> (102.25, 3.525) centre (101.25, 3.525) ccw
  line L62 (101.25, 2.525) -> (89.25, 2.525)
  arc A63 (88.25, 3.525) -> (89.25, 2.525) centre (89.25, 3.525) ccw
  line L63 (88.25, 3.525) -> (88.25, 15.525)
  arc A64 (41.625, 73.675) -> (40.625, 72.675) centre (41.625, 72.675) ccw
  line L64 (41.625, 73.675) -> (53.625, 73.675)
  arc A65 (54.625, 72.675) -> (53.625, 73.675) centre (53.625, 72.675) ccw
  line L65 (54.625, 72.675) -> (54.625, 60.675)
  arc A66 (53.625, 59.675) -> (54.625, 60.675) centre (53.625, 60.675) ccw
  line L66 (53.625, 59.675) -> (41.625, 59.675)
  arc A67 (40.625, 60.675) -> (41.625, 59.675) centre (41.625, 60.675) ccw
  line L67 (40.625, 60.675) -> (40.625, 72.675)
  arc A68 (74.9625, 35.575) -> (73.9625, 34.575) centre (74.9625, 34.575) ccw
  line L68 (74.9625, 35.575) -> (86.9625, 35.575)
  arc A69 (87.9625, 34.575) -> (86.9625, 35.575) centre (86.9625, 34.575) ccw
  line L69 (87.9625, 34.575) -> (87.9625, 22.575)
  arc A70 (86.9625, 21.575) -> (87.9625, 22.575) centre (86.9625, 22.575) ccw
  line L70 (86.9625, 21.575) -> (74.9625, 21.575)
  arc A71 (73.9625, 22.575) -> (74.9625, 21.575) centre (74.9625, 22.575) ccw
  line L71 (73.9625, 22.575) -> (73.9625, 34.575)
  arc A72 (36.8625, 35.575) -> (35.8625, 34.575) centre (36.8625, 34.575) ccw
  line L72 (36.8625, 35.575) -> (48.8625, 35.575)
  arc A73 (49.8625, 34.575) -> (48.8625, 35.575) centre (48.8625, 34.575) ccw
  line L73 (49.8625, 34.575) -> (49.8625, 22.575)
  arc A74 (48.8625, 21.575) -> (49.8625, 22.575) centre (48.8625, 22.575) ccw
  line L74 (48.8625, 21.575) -> (36.8625, 21.575)
  arc A75 (35.8625, 22.575) -> (36.8625, 21.575) centre (36.8625, 22.575) ccw
  line L75 (35.8625, 22.575) -> (35.8625, 34.575)
  arc A76 (227.3625, 16.525) -> (226.3625, 15.525) centre (227.3625, 15.525) ccw
  line L76 (227.3625, 16.525) -> (239.3625, 16.525)
  arc A77 (240.3625, 15.525) -> (239.3625, 16.525) centre (239.3625, 15.525) ccw
  line L77 (240.3625, 15.525) -> (240.3625, 3.525)
  arc A78 (239.3625, 2.525) -> (240.3625, 3.525) centre (239.3625, 3.525) ccw
  line L78 (239.3625, 2.525) -> (227.3625, 2.525)
  arc A79 (226.3625, 3.525) -> (227.3625, 2.525) centre (227.3625, 3.525) ccw
  line L79 (226.3625, 3.525) -> (226.3625, 15.525)
  arc A80 (208.3125, 35.575) -> (207.3125, 34.575) centre (208.3125, 34.575) ccw
  line L80 (208.3125, 35.575) -> (220.3125, 35.575)
  arc A81 (221.3125, 34.575) -> (220.3125, 35.575) centre (220.3125, 34.575) ccw
  line L81 (221.3125, 34.575) -> (221.3125, 22.575)
  arc A82 (220.3125, 21.575) -> (221.3125, 22.575) centre (220.3125, 22.575) ccw
  line L82 (220.3125, 21.575) -> (208.3125, 21.575)
  arc A83 (207.3125, 22.575) -> (208.3125, 21.575) centre (208.3125, 22.575) ccw
  line L83 (207.3125, 22.575) -> (207.3125, 34.575)
  arc A84 (8.2875, 16.525) -> (7.2875, 15.525) centre (8.2875, 15.525) ccw
  line L84 (8.2875, 16.525) -> (20.2875, 16.525)
  arc A85 (21.2875, 15.525) -> (20.2875, 16.525) centre (20.2875, 15.525) ccw
  line L85 (21.2875, 15.525) -> (21.2875, 3.525)
  arc A86 (20.2875, 2.525) -> (21.2875, 3.525) centre (20.2875, 3.525) ccw
  line L86 (20.2875, 2.525) -> (8.2875, 2.525)
  arc A87 (7.2875, 3.525) -> (8.2875, 2.525) centre (8.2875, 3.525) ccw
  line L87 (7.2875, 3.525) -> (7.2875, 15.525)
  arc A88 (51.15, 16.525) -> (50.15, 15.525) centre (51.15, 15.525) ccw
  line L88 (51.15, 16.525) -> (63.15, 16.525)
  arc A89 (64.15, 15.525) -> (63.15, 16.525) centre (63.15, 15.525) ccw
  line L89 (64.15, 15.525) -> (64.15, 3.525)
  arc A90 (63.15, 2.525) -> (64.15, 3.525) centre (63.15, 3.525) ccw
  line L90 (63.15, 2.525) -> (51.15, 2.525)
  arc A91 (50.15, 3.525) -> (51.15, 2.525) centre (51.15, 3.525) ccw
  line L91 (50.15, 3.525) -> (50.15, 15.525)
  arc A92 (198.7875, 54.625) -> (197.7875, 53.625) centre (198.7875, 53.625) ccw
  line L92 (198.7875, 54.625) -> (210.7875, 54.625)
  arc A93 (211.7875, 53.625) -> (210.7875, 54.625) centre (210.7875, 53.625) ccw
  line L93 (211.7875, 53.625) -> (211.7875, 41.625)
  arc A94 (210.7875, 40.625) -> (211.7875, 41.625) centre (210.7875, 41.625) ccw
  line L94 (210.7875, 40.625) -> (198.7875, 40.625)
  arc A95 (197.7875, 41.625) -> (198.7875, 40.625) centre (198.7875, 41.625) ccw
  line L95 (197.7875, 41.625) -> (197.7875, 53.625)
  arc A96 (224.9813, 73.675) -> (223.9813, 72.675) centre (224.9813, 72.675) ccw
  line L96 (224.9813, 73.675) -> (236.9813, 73.675)
  arc A97 (237.9812, 72.675) -> (236.9813, 73.675) centre (236.9813, 72.675) ccw
  line L97 (237.9812, 72.675) -> (237.9813, 60.675)
  arc A98 (236.9813, 59.675) -> (237.9813, 60.675) centre (236.9813, 60.675) ccw
  line L98 (236.9813, 59.675) -> (224.9813, 59.675)
  arc A99 (223.9812, 60.675) -> (224.9813, 59.675) centre (224.9813, 60.675) ccw
  line L99 (223.9812, 60.675) -> (223.9813, 72.675)
  arc A100 (170.2125, 35.575) -> (169.2125, 34.575) centre (170.2125, 34.575) ccw
  line L100 (170.2125, 35.575) -> (182.2125, 35.575)
  arc A101 (183.2125, 34.575) -> (182.2125, 35.575) centre (182.2125, 34.575) ccw
  line L101 (183.2125, 34.575) -> (183.2125, 22.575)
  arc A102 (182.2125, 21.575) -> (183.2125, 22.575) centre (182.2125, 22.575) ccw
  line L102 (182.2125, 21.575) -> (170.2125, 21.575)
  arc A103 (169.2125, 22.575) -> (170.2125, 21.575) centre (170.2125, 22.575) ccw
  line L103 (169.2125, 22.575) -> (169.2125, 34.575)
  arc A104 (127.35, 16.525) -> (126.35, 15.525) centre (127.35, 15.525) ccw
  line L104 (127.35, 16.525) -> (139.35, 16.525)
  arc A105 (140.35, 15.525) -> (139.35, 16.525) centre (139.35, 15.525) ccw
  line L105 (140.35, 15.525) -> (140.35, 3.525)
  arc A106 (139.35, 2.525) -> (140.35, 3.525) centre (139.35, 3.525) ccw
  line L106 (139.35, 2.525) -> (127.35, 2.525)
  arc A107 (126.35, 3.525) -> (127.35, 2.525) centre (127.35, 3.525) ccw
  line L107 (126.35, 3.525) -> (126.35, 15.525)
  arc A108 (113.0625, 35.575) -> (112.0625, 34.575) centre (113.0625, 34.575) ccw
  line L108 (113.0625, 35.575) -> (125.0625, 35.575)
  arc A109 (126.0625, 34.575) -> (125.0625, 35.575) centre (125.0625, 34.575) ccw
  line L109 (126.0625, 34.575) -> (126.0625, 22.575)
  arc A110 (125.0625, 21.575) -> (126.0625, 22.575) centre (125.0625, 22.575) ccw
  line L110 (125.0625, 21.575) -> (113.0625, 21.575)
  arc A111 (112.0625, 22.575) -> (113.0625, 21.575) centre (113.0625, 22.575) ccw
  line L111 (112.0625, 22.575) -> (112.0625, 34.575)
  arc A112 (84.4875, 54.625) -> (83.4875, 53.625) centre (84.4875, 53.625) ccw
  line L112 (84.4875, 54.625) -> (96.4875, 54.625)
  arc A113 (97.4875, 53.625) -> (96.4875, 54.625) centre (96.4875, 53.625) ccw
  line L113 (97.4875, 53.625) -> (97.4875, 41.625)
  arc A114 (96.4875, 40.625) -> (97.4875, 41.625) centre (96.4875, 41.625) ccw
  line L114 (96.4875, 40.625) -> (84.4875, 40.625)
  arc A115 (83.4875, 41.625) -> (84.4875, 40.625) centre (84.4875, 41.625) ccw
  line L115 (83.4875, 41.625) -> (83.4875, 53.625)
  arc A116 (146.4, 16.525) -> (145.4, 15.525) centre (146.4, 15.525) ccw
  line L116 (146.4, 16.525) -> (158.4, 16.525)
  arc A117 (159.4, 15.525) -> (158.4, 16.525) centre (158.4, 15.525) ccw
  line L117 (159.4, 15.525) -> (159.4, 3.525)
  arc A118 (158.4, 2.525) -> (159.4, 3.525) centre (158.4, 3.525) ccw
  line L118 (158.4, 2.525) -> (146.4, 2.525)
  arc A119 (145.4, 3.525) -> (146.4, 2.525) centre (146.4, 3.525) ccw
  line L119 (145.4, 3.525) -> (145.4, 15.525)
  arc A120 (189.2625, 35.575) -> (188.2625, 34.575) centre (189.2625, 34.575) ccw
  line L120 (189.2625, 35.575) -> (201.2625, 35.575)
  arc A121 (202.2625, 34.575) -> (201.2625, 35.575) centre (201.2625, 34.575) ccw
  line L121 (202.2625, 34.575) -> (202.2625, 22.575)
  arc A122 (201.2625, 21.575) -> (202.2625, 22.575) centre (201.2625, 22.575) ccw
  line L122 (201.2625, 21.575) -> (189.2625, 21.575)
  arc A123 (188.2625, 22.575) -> (189.2625, 21.575) centre (189.2625, 22.575) ccw
  line L123 (188.2625, 22.575) -> (188.2625, 34.575)
  circle A124 centre (220.025, 66.675) radius 1.25
  circle A125 centre (245.269, 9.525) radius 1.25
  arc A126 (203.55, 16.525) -> (202.55, 15.525) centre (203.55, 15.525) ccw
  line L124 (203.55, 16.525) -> (215.55, 16.525)
  arc A127 (216.55, 15.525) -> (215.55, 16.525) centre (215.55, 15.525) ccw
  line L125 (216.55, 15.525) -> (216.55, 3.525)
  arc A128 (215.55, 2.525) -> (216.55, 3.525) centre (215.55, 3.525) ccw
  line L126 (215.55, 2.525) -> (203.55, 2.525)
  arc A129 (202.55, 3.525) -> (203.55, 2.525) centre (203.55, 3.525) ccw
  line L127 (202.55, 3.525) -> (202.55, 15.525)
  arc A130 (131.5375, 60.675) -> (132.5375, 59.675) centre (132.5375, 60.675) ccw
  line L128 (131.5375, 60.675) -> (131.5375, 72.675)
  arc A131 (132.5375, 73.675) -> (131.5375, 72.675) centre (132.5375, 72.675) ccw
  line L129 (132.5375, 73.675) -> (162.7375, 73.675)
  arc A132 (163.7375, 72.675) -> (162.7375, 73.675) centre (162.7375, 72.675) ccw
  line L130 (163.7375, 72.675) -> (163.7375, 60.675)
  arc A133 (162.7375, 59.675) -> (163.7375, 60.675) centre (162.7375, 60.675) ccw
  line L131 (162.7375, 59.675) -> (132.5375, 59.675)
  arc A134 (5.3312, 41.625) -> (6.3312, 40.625) centre (6.3312, 41.625) ccw
  line L132 (5.3312, 41.625) -> (5.3313, 53.625)
  arc A135 (6.3312, 54.625) -> (5.3312, 53.625) centre (6.3312, 53.625) ccw
  line L133 (6.3312, 54.625) -> (36.5313, 54.625)
  arc A136 (37.5312, 53.625) -> (36.5313, 54.625) centre (36.5313, 53.625) ccw
  line L134 (37.5312, 53.625) -> (37.5313, 41.625)
  arc A137 (36.5313, 40.625) -> (37.5312, 41.625) centre (36.5313, 41.625) ccw
  line L135 (36.5313, 40.625) -> (6.3312, 40.625)
  arc A138 (141.6375, 54.625) -> (140.6375, 53.625) centre (141.6375, 53.625) ccw
  line L136 (141.6375, 54.625) -> (153.6375, 54.625)
  arc A139 (154.6375, 53.625) -> (153.6375, 54.625) centre (153.6375, 53.625) ccw
  line L137 (154.6375, 53.625) -> (154.6375, 41.625)
  arc A140 (153.6375, 40.625) -> (154.6375, 41.625) centre (153.6375, 41.625) ccw
  line L138 (153.6375, 40.625) -> (141.6375, 40.625)
  arc A141 (140.6375, 41.625) -> (141.6375, 40.625) centre (141.6375, 41.625) ccw
  line L139 (140.6375, 41.625) -> (140.6375, 53.625)
  arc A142 (108.3, 16.525) -> (107.3, 15.525) centre (108.3, 15.525) ccw
  line L140 (108.3, 16.525) -> (120.3, 16.525)
  arc A143 (121.3, 15.525) -> (120.3, 16.525) centre (120.3, 15.525) ccw
  line L141 (121.3, 15.525) -> (121.3, 3.525)
  arc A144 (120.3, 2.525) -> (121.3, 3.525) centre (120.3, 3.525) ccw
  line L142 (120.3, 2.525) -> (108.3, 2.525)
  arc A145 (107.3, 3.525) -> (108.3, 2.525) centre (108.3, 3.525) ccw
  line L143 (107.3, 3.525) -> (107.3, 15.525)
  arc A146 (179.7375, 54.625) -> (178.7375, 53.625) centre (179.7375, 53.625) ccw
  line L144 (179.7375, 54.625) -> (191.7375, 54.625)
  arc A147 (192.7375, 53.625) -> (191.7375, 54.625) centre (191.7375, 53.625) ccw
  line L145 (192.7375, 53.625) -> (192.7375, 41.625)
  arc A148 (191.7375, 40.625) -> (192.7375, 41.625) centre (191.7375, 41.625) ccw
  line L146 (191.7375, 40.625) -> (179.7375, 40.625)
  arc A149 (178.7375, 41.625) -> (179.7375, 40.625) centre (179.7375, 41.625) ccw
  line L147 (178.7375, 41.625) -> (178.7375, 53.625)
  arc A150 (217.8375, 54.625) -> (216.8375, 53.625) centre (217.8375, 53.625) ccw
  line L148 (217.8375, 54.625) -> (229.8375, 54.625)
  arc A151 (230.8375, 53.625) -> (229.8375, 54.625) centre (229.8375, 53.625) ccw
  line L149 (230.8375, 53.625) -> (230.8375, 41.625)
  arc A152 (229.8375, 40.625) -> (230.8375, 41.625) centre (229.8375, 41.625) ccw
  line L150 (229.8375, 40.625) -> (217.8375, 40.625)
  arc A153 (216.8375, 41.625) -> (217.8375, 40.625) centre (217.8375, 41.625) ccw
  line L151 (216.8375, 41.625) -> (216.8375, 53.625)
  arc A154 (122.5875, 54.625) -> (121.5875, 53.625) centre (122.5875, 53.625) ccw
  line L152 (122.5875, 54.625) -> (134.5875, 54.625)
  arc A155 (135.5875, 53.625) -> (134.5875, 54.625) centre (134.5875, 53.625) ccw
  line L153 (135.5875, 53.625) -> (135.5875, 41.625)
  arc A156 (134.5875, 40.625) -> (135.5875, 41.625) centre (134.5875, 41.625) ccw
  line L154 (134.5875, 40.625) -> (122.5875, 40.625)
  arc A157 (121.5875, 41.625) -> (122.5875, 40.625) centre (122.5875, 41.625) ccw
  line L155 (121.5875, 41.625) -> (121.5875, 53.625)
  arc A158 (160.6875, 54.625) -> (159.6875, 53.625) centre (160.6875, 53.625) ccw
  line L156 (160.6875, 54.625) -> (172.6875, 54.625)
  arc A159 (173.6875, 53.625) -> (172.6875, 54.625) centre (172.6875, 53.625) ccw
  line L157 (173.6875, 53.625) -> (173.6875, 41.625)
  arc A160 (172.6875, 40.625) -> (173.6875, 41.625) centre (172.6875, 41.625) ccw
  line L158 (172.6875, 40.625) -> (160.6875, 40.625)
  arc A161 (159.6875, 41.625) -> (160.6875, 40.625) centre (160.6875, 41.625) ccw
  line L159 (159.6875, 41.625) -> (159.6875, 53.625)
  arc A162 (103.5375, 54.625) -> (102.5375, 53.625) centre (103.5375, 53.625) ccw